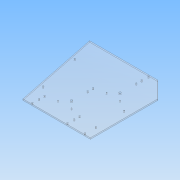
# Autodesk Inventor part: Top_Separator Backboard 3 Lanes
Saved by Autodesk Inventor 2018.1 (Build 221171000, 171)
## iProperties
Created: 2019-03-20
Part Number: Top_Separator Backboard 3 Lanes
Material: PMMA Plastic
Document SubType Name: Modeling
Designer: James
Density: 1.188 g/cm^3
Appearance: Polycarbonate - Clear
Author: James
Autodesk Inventor part; units mm, degrees
ref_plane "YZ Plane" through (0, 0, 0) normal (1, 0, 0) x (0, 1, 0)
ref_plane "XZ Plane" through (0, 0, 0) normal (0, 1, 0) x (-1, 0, 0)
ref_plane "XY Plane" through (0, 0, 0) normal (0, 0, 1) x (1, 0, 0)
sketch "Sketch1" plane through (0, 0, 0) normal (0, 0, 1) x (1, 0, 0)
  line L0 (0, 0) -> (-63.0702, 310)
  line L1 (-63.0702, 310) -> (250, 310)
  line L2 (250, 310) -> (250, 0)
  line L3 (250, 0) -> (0, 0)
  dimension "d0" = 310
  dimension "d1" = 78.5
  dimension "d2" = 250
  constraints: 8 end point, 2 perpendicular, 1 horizontal
  measures "d0" distance of L1.end L2.end
  measures "d1" angle of L3 L0
  measures "d2" distance of L2.end L0.start
extrude "Extrusion1" add sketch "Sketch1" along normal blind 5
sketch "Sketch2" plane through (0, 0, 5) normal (0, 0, 1) x (1, 0, 0)
  line L0 (0, 0) -> (250, 0) projected
  point P0 (160, 280)
  point P1 (160, 260)
  point P2 (95, 165)
  point P3 (95, 145)
  point P4 (225, 150)
  point P5 (225, 45)
  point P6 (30, 50)
  point P7 (30, 30)
  point P8 (160, 50)
  point P9 (160, 30)
  point P10 (160, 305)
  point P11 (30, 5)
  point P12 (160, 5)
  point P13 (225, 5)
  dimension "d7" = 20
  dimension "d15" = 25
  dimension "d20" = 5
  dimension "d21" = 30
  dimension "d30" = 130
  dimension "d32" = 65
  dimension "d36" = 65
  dimension "d92" = 25
  dimension "d93" = 20
  dimension "d94" = 95
  dimension "d95" = 20
  dimension "d96" = 95
  dimension "d97" = 105
  dimension "d98" = 130
  dimension "d99" = 15
  constraints: 9 vertical alignment, 4 horizontal alignment
  measures "d7" distance of point (160, 260) point (160, 280)
  measures "d15" distance of point (160, 305) point (160, 280)
  measures "d20" distance from line of L0 point (30, 5)
  measures "d21" horizontal distance of point (30, 5) L0.start
  measures "d30" distance of point (160, 5) point (30, 5)
  measures "d32" horizontal distance of point (30, 50) point (95, 145)
  measures "d36" horizontal distance of point (95, 165) point (160, 260)
  measures "d92" distance of point (160, 30) point (160, 5)
  measures "d93" distance of point (160, 30) point (160, 50)
  measures "d94" vertical distance of point (95, 165) point (160, 260)
  measures "d95" distance of point (95, 145) point (95, 165)
  measures "d96" vertical distance of point (160, 50) point (95, 145)
  measures "d97" distance of point (225, 150) point (225, 45)
  measures "d98" horizontal distance of point (225, 45) point (95, 165)
  measures "d99" vertical distance of point (225, 150) point (95, 165)
hole "Hole1" at (160, 280, 5) at (160, 260, 5) at (95, 165, 5) at (95, 145, 5) at (225, 150, 5) at (225, 45, 5) at (30, 50, 5) at (30, 30, 5) at (160, 50, 5) at (160, 30, 5) at (160, 305, 5) at (30, 5, 5) at (160, 5, 5) at (225, 5, 5) direction (0, 0, -1) diameter 4.5 end through all clearance for "Flat Head Machine Screw" size "M4" standard "Ansi Metric M Profile"
sketch "Sketch3" plane through (0, 0, 5) normal (0, 0, 1) x (1, 0, 0)
  circle A0 centre (30, 5) radius 2.25 projected
  circle A1 centre (160, 30) radius 2.25 projected
  circle A2 centre (30, 30) radius 2.25 projected
  circle A3 centre (225, 45) radius 2.25 projected
  circle A4 centre (95, 145) radius 2.25 projected
  circle A5 centre (160, 260) radius 2.25 projected
  circle A6 centre (160, 280) radius 2.25 projected
  circle A7 centre (95, 165) radius 2.25 projected
  circle A8 centre (225, 150) radius 2.25 projected
  circle A9 centre (30, 50) radius 2.25 projected
  circle A10 centre (160, 50) radius 2.25 projected
  circle A11 centre (160, 5) radius 2.25 projected
  line L0 (-63.0702, 310) -> (0, 0) projected
  line L1 (0, 0) -> (250, 0) projected
  line L2 (250, 0) -> (250, 310) projected
  line L3 (250, 310) -> (-63.0702, 310) projected
  point P0 (160, 200)
  point P1 (95, 85)
  dimension "d37" = 60
  dimension "d89" = 60
  constraints: 2 vertical alignment
  measures "d37" distance of A5.centre point (160, 200)
  measures "d89" distance of A4.centre point (95, 85)
hole "Hole2" at (160, 200, 5) at (95, 85, 5) direction (0, 0, -1) diameter 7 end through all
sketch "Sketch4" plane through (0, 0, 5) normal (0, 0, 1) x (1, 0, 0)
  circle A0 centre (95, 85) radius 3.5 projected
  circle A1 centre (160, 200) radius 3.5 projected
  circle A2 centre (30, 5) radius 2.25 projected
  circle A3 centre (160, 30) radius 2.25 projected
  circle A4 centre (30, 30) radius 2.25 projected
  circle A5 centre (225, 45) radius 2.25 projected
  circle A6 centre (95, 145) radius 2.25 projected
  circle A7 centre (160, 260) radius 2.25 projected
  circle A8 centre (160, 280) radius 2.25 projected
  circle A9 centre (95, 165) radius 2.25 projected
  circle A10 centre (225, 150) radius 2.25 projected
  circle A11 centre (30, 50) radius 2.25 projected
  circle A12 centre (160, 50) radius 2.25 projected
  circle A13 centre (160, 5) radius 2.25 projected
  line L0 (-63.0702, 310) -> (0, 0) projected
  line L1 (0, 0) -> (250, 0) projected
  line L2 (250, 0) -> (250, 310) projected
  line L3 (250, 310) -> (-63.0702, 310) projected
  point P0 (185, 175)
  point P1 (135, 175)
  point P2 (70, 60)
  point P3 (120, 60)
  dimension "d46" = 25
  dimension "d47" = 25
  dimension "d48" = 50
  dimension "d49" = 50
  dimension "d50" = 25
  constraints: 2 horizontal alignment
  measures "d46" horizontal distance of A1.centre point (135, 175)
  measures "d47" horizontal distance of A1.centre point (135, 175)
  measures "d48" distance of point (185, 175) point (135, 175)
  measures "d49" distance of point (70, 60) point (120, 60)
  measures "d50" horizontal distance of A0.centre point (70, 60)
hole "Hole3" at (185, 175, 5) at (135, 175, 5) at (70, 60, 5) at (120, 60, 5) direction (0, 0, -1) diameter 3.4 end through all clearance for "Flat Head Machine Screw" size "M3" standard "Ansi Metric M Profile"
chamfer "Chamfer1" distance 60 angle 45 1 edges at (250, 310, 2.5)
sketch "Sketch5" plane through (0, 0, 5) normal (0, 0, 1) x (1, 0, 0)
  line L0 (-63.0702, 310) -> (0, 0) projected
  line L1 (190, 310) -> (-63.0702, 310) projected
  line L2 (0, 0) -> (250, 0) projected
  point P0 (-33.0207, 225)
  point P1 (-3.1155, 78.0113)
  dimension "d64" = 12.5
  dimension "d65" = 12.5
  dimension "d66" = 150
  dimension "d67" = 85
  dimension "d68" = 78.0113
  measures "d64" distance from line of point (-33.021, 225) L0
  measures "d65" distance from line of L0 point (-3.115, 78.011)
  measures "d66" distance of point (-33.021, 225) point (-3.115, 78.011)
  measures "d67" distance from line of L1 point (-33.021, 225)
  measures "d68" distance from line of L2 point (-3.115, 78.011)
hole "Hole4" at (-33.0207, 225, 5) at (-3.1155, 78.0113, 5) direction (0, 0, -1) diameter 4.5 end through all clearance for "Flat Head Machine Screw" size "M4" standard "Ansi Metric M Profile"
sketch "Sketch6" plane through (0, 0, 5) normal (0, 0, 1) x (1, 0, 0)
  circle A0 centre (-33.0207, 225) radius 2.25 projected
  circle A1 centre (-3.1155, 78.0113) radius 2.25 projected
  line L0 (190, 310) -> (250, 250) projected
  line L1 (190, 310) -> (-63.0702, 310) projected
  line L2 (-63.0702, 310) -> (0, 0) projected
  line L3 (0, 0) -> (250, 0) projected
  line L4 (250, 0) -> (250, 250) projected
  circle A2 centre (70, 60) radius 1.7 projected
  circle A3 centre (185, 175) radius 1.7 projected
  circle A4 centre (135, 175) radius 1.7 projected
  circle A5 centre (120, 60) radius 1.7 projected
  circle A6 centre (95, 85) radius 3.5 projected
  circle A7 centre (160, 200) radius 3.5 projected
  circle A8 centre (30, 5) radius 2.25 projected
  circle A9 centre (160, 30) radius 2.25 projected
  circle A10 centre (30, 30) radius 2.25 projected
  circle A11 centre (225, 45) radius 2.25 projected
  circle A12 centre (95, 145) radius 2.25 projected
  circle A13 centre (95, 165) radius 2.25 projected
  circle A14 centre (225, 150) radius 2.25 projected
  circle A15 centre (30, 50) radius 2.25 projected
  circle A16 centre (160, 50) radius 2.25 projected
  circle A17 centre (160, 5) radius 2.25 projected
  point P0 (95.4041, 170)
  point P1 (115, 174)
  point P2 (205, 174)
  point P3 (224.5959, 170)
  dimension "d76" = 20
  dimension "d77" = 4
  dimension "d78" = 20
  dimension "d79" = 45
  dimension "d80" = 26
  dimension "d81" = 45
  constraints: 2 horizontal alignment
  measures "d76" distance of point (115, 174) point (95.404, 170)
  measures "d77" vertical distance of point (95.404, 170) point (115, 174)
  measures "d78" distance of point (224.596, 170) point (205, 174)
  measures "d79" horizontal distance of A7.centre point (115, 174)
  measures "d80" vertical distance of A7.centre point (115, 174)
  measures "d81" horizontal distance of point (205, 174) A7.centre
hole "Hole5" [suppressed]
equation "\"d7\" = d5"
equation "\"d32\" = 0.5 * d30"
equation "\"d36\" = d32"
equation "\"d93\" = d7"
equation "\"d98\" = 2 * d36"
equation "\"d48\" = 2 * d47"
equation "\"d49\" = d48"
equation "\"d50\" = 0.5 * d49"
equation "\"d65\" = d64"
equation "\"d78\" = d76"
equation "\"d81\" = d79"
equation "\"d5\" = d6"
equation "\"d6\" = 20"
body "Solid1"
